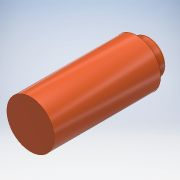
# Autodesk Inventor part: Pok X-Carriage Bottom Support
Saved by Autodesk Inventor 2018.2 (Build 222227000, 227)
## iProperties
Created: 2018-02-07
Part Number: Pok X-Carriage Bottom Support
Material: ABS Plastic
Document SubType Name: Modeling
Designer: Moochster
Density: 1.06 g/cm^3
Appearance: Smooth - Light Orange
Author: Moochster
Autodesk Inventor part; units mm, degrees
ref_plane "YZ Plane" through (0, 0, 0) normal (1, 0, 0) x (0, 1, 0)
ref_plane "XZ Plane" through (0, 0, 0) normal (0, 1, 0) x (-1, 0, 0)
ref_plane "XY Plane" through (0, 0, 0) normal (0, 0, 1) x (1, 0, 0)
sketch "Sketch1" plane through (0, 0, 0) normal (0, 0, 1) x (1, 0, 0)
  line L0 (0, 0) -> (0, 20)
  line L1 (0, 20) -> (2.85, 20)
  line L2 (2.85, 20) -> (2.85, 17.9)
  line L3 (2.85, 17.9) -> (4, 17.9)
  line L4 (4, 17.9) -> (4, 0)
  line L5 (4, 0) -> (0, 0)
  dimension "d0" = 8
  dimension "d1" = 5.7
  dimension "d2" = 2.1
  dimension "d3" = 20
  constraints: 12 end point, 4 perpendicular, 1 horizontal, 1 vertical
  measures "d0" diameter of L4 L0
  measures "d1" diameter of L2 L0
  measures "d2" distance of L1.end L2.end
  measures "d3" distance of L0.start L0.end
revolve "Revolution1" add sketch "Sketch1" angle 360 about axis through (0, 0, 0) along (0, 1, 0)
fillet "Fillet1" radius 0.3 1 edges at (-2.85, 20, 0)
body "Solid1"
